# Autodesk Inventor part: PCAP_1210
Saved by Autodesk Inventor 2015 SP1 (Build 190203100, 203)
## iProperties
Created: 2015-06-25
Part Number: PCAP_1210
Material: Generic
Document SubType Name: Modeling
Designer: Patrick
Density: 1 g/cm^3
Appearance: CAP_1210, PCAP_1210
Author: Patrick
Autodesk Inventor part; units mm, degrees
ref_plane "YZ Plane" through (0, 0, 0) normal (1, 0, 0) x (0, 1, 0)
ref_plane "XZ Plane" through (0, 0, 0) normal (0, 1, 0) x (-1, 0, 0)
ref_plane "XY Plane" through (0, 0, 0) normal (0, 0, 1) x (1, 0, 0)
sketch "CAP_1210, PCAP_1210_216" plane through (0, 0, 0) normal (0, 0, 1) x (1, 0, 0)
  line L0 (-2.275, -1.44) -> (-2.275, 1.53)
  line L1 (-2.275, 1.53) -> (2.275, 1.53)
  line L2 (2.275, 1.53) -> (2.275, -1.44)
  line L3 (2.275, -1.44) -> (-2.275, -1.44)
  constraints: 8 end point
extrude "Extrusion1" add sketch "CAP_1210, PCAP_1210_216" along normal blind 1
body "Solid1"
